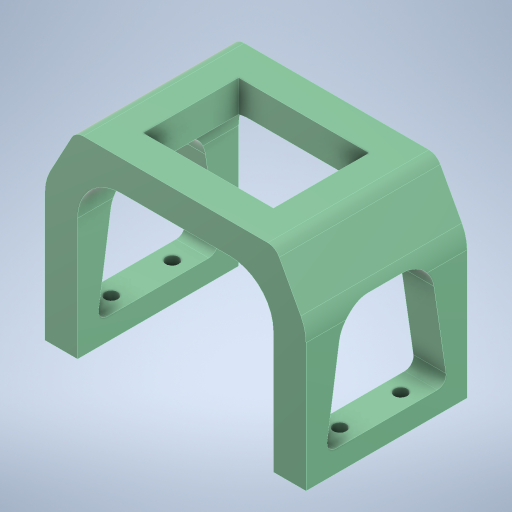
# Autodesk Inventor part: switchHandle
Saved by Autodesk Inventor 2023 (Build 270158000, 158)
## iProperties
Created: 2023-08-24
Part Number: switchHandle
Material: Generic
Document SubType Name: Modeling
Designer: Dawid
Density: 1 g/cm^3
Appearance: Smooth - Dark Sea Green
Author: Dawid
Autodesk Inventor part; units mm, degrees
ref_plane "YZ Plane" through (0, 0, 0) normal (1, 0, 0) x (0, 1, 0)
ref_plane "XZ Plane" through (0, 0, 0) normal (0, 1, 0) x (-1, 0, 0)
ref_plane "XY Plane" through (0, 0, 0) normal (0, 0, 1) x (1, 0, 0)
sketch "Sketch1" plane through (0, 0, 0) normal (0, 1, 0) x (-1, 0, 0)
  line L0 (22.5, 18.5) -> (-22.5, 18.5)
  line L1 (-22.5, 18.5) -> (-22.5, -18.5)
  line L2 (-22.5, -18.5) -> (22.5, -18.5)
  line L3 (22.5, -18.5) -> (22.5, 18.5)
  line L4 (22.5, 18.5) -> (-22.5, -18.5) construction
  line L5 (-22.5, 18.5) -> (22.5, -18.5) construction
  line L6 (30, 18.5) -> (-30, 18.5)
  line L7 (-30, 18.5) -> (-30, -18.5)
  line L8 (-30, -18.5) -> (30, -18.5)
  line L9 (30, -18.5) -> (30, 18.5)
  line L10 (30, 18.5) -> (-30, -18.5) construction
  line L11 (-30, 18.5) -> (30, -18.5) construction
  point P0 (0, 0)
  dimension "d0" = 45
  dimension "d1" = 37
  dimension "d2" = 60
  dimension "d3" = 37
  constraints: 24 end point, 4 midpoint, 4 parallel, 2 horizontal, 2 perpendicular
  measures "d0" distance of L2.end L1.end
  measures "d1" distance of L1.end L0.end
  measures "d2" distance of L8.end L7.end
  measures "d3" distance of L7.end L6.end
extrude "Extrusion1" add sketch "Sketch1" along normal blind 45 contours L6 L9 L8 L3 | L1 L8 L7 L6
sketch "Sketch2" plane through (0, 45, 0) normal (0, 1, 0) x (1, 0, 0)
  line L0 (-30, -18.5) -> (-22.5, -18.5) projected
  line L1 (30, 18.5) -> (22.5, 18.5) projected
  line L2 (-30, -18.5) -> (30, -18.5)
  line L3 (30, -18.5) -> (30, 18.5)
  line L4 (30, 18.5) -> (-30, 18.5)
  line L5 (-30, 18.5) -> (-30, -18.5)
  point P0 (0, 0)
  constraints: 8 end point, 2 parallel, 1 horizontal, 1 perpendicular
extrude "Extrusion2" add sketch "Sketch2" against normal blind 7
sketch "Sketch3" plane through (0, 45, 0) normal (0, 1, 0) x (1, 0, 0)
  line L0 (-15, -11) -> (15, -11)
  line L1 (15, -11) -> (15, 11)
  line L2 (15, 11) -> (-15, 11)
  line L3 (-15, 11) -> (-15, -11)
  line L4 (-15, -11) -> (15, 11) construction
  line L5 (15, -11) -> (-15, 11) construction
  point P0 (0, 0)
  dimension "d8" = 30
  dimension "d9" = 22
  constraints: 12 end point, 2 midpoint, 2 parallel, 1 horizontal, 1 perpendicular
  measures "d8" distance of L2.end L1.end
  measures "d9" distance of L1.end L0.end
extrude "Extrusion3" cut sketch "Sketch3" against normal blind 10
sketch "Sketch6" plane through (30, 0, 18.5) normal (1, 0, 0) x (0, 0, -1)
  line L0 (37, 0) -> (0, 0) projected
  line L1 (0, 0) -> (0, 5)
  line L2 (0, 0) -> (0, 38) projected
  line L3 (0, 5) -> (37, 5)
  line L4 (37, 0) -> (37, 38) projected
  line L5 (0, 5) -> (18.5, 5)
  line L6 (18.5, 5) -> (32.5, 5)
  line L7 (32.5, 5) -> (4.5, 5)
  line L8 (18.5, 5) -> (18.5, 32)
  line L9 (18.5, 32) -> (28.5, 32)
  line L10 (28.5, 32) -> (8.5, 32)
  line L11 (8.5, 32) -> (4.5, 5)
  line L12 (32.5, 5) -> (28.5, 32)
  point P0 (18.5, 0)
  point P1 (4.5, 5)
  dimension "d12" = 5
  dimension "d13" = 14
  dimension "d14" = 28
  dimension "d15" = 27
  dimension "d16" = 10
  dimension "d17" = 20
  constraints: 20 end point, 5 point on line, 3 perpendicular, 1 midpoint
  measures "d12" distance of L0.end L1.end
  measures "d13" distance of L5.end L6.end
  measures "d14" distance of L6.end L7.end
  measures "d15" distance of L5.end L8.end
  measures "d16" distance of L8.end L9.end
  measures "d17" distance of L9.end L10.end
extrude "Extrusion4" cut sketch "Sketch6" against normal blind 100 contours L3 L8 L9 L12 | L11 L10 L8 L3
sketch "Sketch7" plane through (0, 0, 0) normal (0, -1, 0) x (1, 0, 0)
  line L0 (30, 18.5) -> (30, -18.5) projected
  line L1 (30, 0) -> (22.5, 0)
  line L2 (22.5, -18.5) -> (22.5, 18.5) projected
  line L3 (30, 0) -> (26.25, 0)
  line L4 (26.25, 0) -> (26.25, -18.5)
  line L5 (30, -18.5) -> (-30, -18.5) projected
  line L6 (26.25, -18.5) -> (26.25, -9.25)
  line L7 (26.25, 0) -> (26.25, 18.5)
  line L8 (-30, 18.5) -> (30, 18.5) projected
  line L9 (26.25, 18.5) -> (26.25, 9.25)
  line L10 (26.25, -18.5) -> (26.25, -9.25)
  line L11 (-30, -18.5) -> (-30, 18.5) projected
  line L12 (-22.5, -18.5) -> (22.5, -18.5) projected
  line L13 (-30, -18.5) -> (-22.5, -18.5)
  line L14 (-22.5, -18.5) -> (-26.25, -18.5)
  line L15 (-26.25, -18.5) -> (-26.25, 18.5)
  line L16 (-26.25, 0) -> (-26.25, 7)
  line L17 (-26.25, 7) -> (-26.25, -7)
  line L18 (26.25, 0) -> (26.25, -7)
  line L19 (26.25, -7) -> (26.25, 7)
  circle A0 centre (26.25, 7) radius 1.5
  circle A1 centre (26.25, -7) radius 1.5
  circle A2 centre (-26.25, -7) radius 1.5
  circle A3 centre (-26.25, 7) radius 1.5
  point P0 (0, 0)
  dimension "d34" = 7
  dimension "d35" = 14
  dimension "d36" = 7
  dimension "d37" = 14
  dimension "d38" = 3
  dimension "d39" = 3
  dimension "d40" = 3
  dimension "d41" = 3
  constraints: 28 end point, 8 point on line, 7 midpoint, 4 centre point, 4 coincident, 2 perpendicular, 1 collinear, 1 horizontal
  measures "d34" distance of L16.start L16.end
  measures "d35" distance of L16.end L17.end
  measures "d36" distance of L3.end L18.end
  measures "d37" distance of L18.end L19.end
  measures "d38" diameter of A0
  measures "d39" diameter of A1
  measures "d40" diameter of A2
  measures "d41" diameter of A3
extrude "Extrusion5" cut sketch "Sketch7" against normal blind 10 contours A1 L4 | L4 A1 | A0 L7 | L7 A0 | A3 L15 | L15 A3 | A2 L15 | L15 A2
fillet "Fillet1" radius 10 2 edges at (22.5, 38, 0) (-22.5, 38, 0)
fillet "Fillet2" radius 7 4 edges at (25.8326, 32, 10) (-25.8326, 32, 10) (-25.8326, 32, -10) (25.8326, 32, -10)
chamfer "Chamfer1" distance 7 distance2 13 2 edges at (30, 45, 0) (-30, 45, 0) measured on face at (-29.5, 45, 0) measured on face at (29.5, 45, 0)
fillet "Fillet3" radius 3 2 edges at (-23.0001, 45, 0) (23.0001, 45, 0)
fillet "Fillet4" radius 10 2 edges at (30, 32.0001, 0) (-30, 32.0001, 0)
fillet "Fillet5" radius 2 4 edges at (26.25, 5, 14) (-26.25, 5, 14) (26.25, 5, -14) (-26.25, 5, -14)
body "Solid1"
